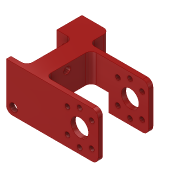
# Autodesk Inventor part: Odometry_Holder with motor clearance
Saved by Autodesk Inventor 2020 (Build 240168000, 168)
## iProperties
Created: 2019-06-02
Part Number: Odometry_Holder with motor clearance
Material: Generic
Document SubType Name: Modeling
Designer: ishaa
Density: 1 g/cm^3
Appearance: Default
Author: ishaa
Autodesk Inventor part; units mm, degrees
ref_plane "YZ Plane" through (0, 0, 0) normal (1, 0, 0) x (0, 1, 0)
ref_plane "XZ Plane" through (0, 0, 0) normal (0, 1, 0) x (-1, 0, 0)
ref_plane "XY Plane" through (0, 0, 0) normal (0, 0, 1) x (1, 0, 0)
sketch "Sketch1" plane through (0, 0, 0) normal (0, 1, 0) x (-1, 0, 0)
  line L0 (-8.3746, 16.5585) -> (42.4254, 16.5585)
  line L1 (42.4254, 16.5585) -> (42.4254, 14.0185)
  line L2 (42.4254, 14.0185) -> (33.5354, 14.0185)
  line L3 (33.5354, 14.0185) -> (33.5354, -11.3815)
  line L4 (33.5354, -11.3815) -> (42.4254, -11.3815)
  line L5 (42.4254, -11.3815) -> (42.4254, -13.9215)
  line L6 (42.4254, -13.9215) -> (-8.3746, -13.9215)
  line L7 (-8.3746, 16.5585) -> (-8.3746, 14.0185)
  line L8 (-8.3746, 14.0185) -> (23.3754, 14.0185)
  line L9 (23.3754, 14.0185) -> (23.3754, -11.3815)
  line L10 (23.3754, -11.3815) -> (-8.3746, -11.3815)
  line L11 (-8.3746, -11.3815) -> (-8.3746, -13.9215)
  point P0 (0, 0)
  dimension "d0" = 30.48
  dimension "d1" = 2.54
  dimension "d2" = 2.54
  dimension "d4" = 2.54
  dimension "d5" = 2.54
  dimension "d6" = 8.89
  dimension "d7" = 50.8
  dimension "d8" = 31.75
  constraints: 24 end point, 9 perpendicular, 3 point on line, 1 horizontal, 1 vertical
  measures "d0" distance between parallel lines of L0 L6
  measures "d1" distance between parallel lines of L8 L0
  measures "d2" distance between parallel lines of L6 L10
  measures "d4" distance between parallel lines of L2 L0
  measures "d5" distance between parallel lines of L6 L4
  measures "d6" distance of L1.end L2.end
  measures "d7" distance of L0.start L0.end
  measures "d8" distance of L7.end L8.end
extrude "Extrusion1" add sketch "Sketch1" along normal blind 25.4
sketch "Sketch4" plane through (8.3746, 0, -13.9215) normal (0, 0, -1) x (-1, 0, 0)
  line L0 (50.8, 0) -> (0, 0) projected
  line L1 (50.8, 0) -> (50.8, 25.4) projected
  line L2 (0, 25.4) -> (50.8, 25.4) projected
  line L3 (50.8, 25.4) -> (41.91, 25.4)
  line L4 (41.91, 25.4) -> (41.91, 0)
  line L5 (41.91, 0) -> (50.8, 0)
  line L6 (50.8, 0) -> (50.8, 25.4)
  point P0 (8.3746, 0)
  dimension "d56" = 8.89
  constraints: 8 end point, 2 parallel, 1 horizontal, 1 perpendicular, 1 point on line
  measures "d56" distance of L5.end L4.end
extrude "Extrusion3" add sketch "Sketch4" along normal blind 11.43
sketch "Sketch5" plane through (-42.4254, 0, 16.5585) normal (0, 0, 1) x (1, 0, 0)
  line L0 (50.8, 0) -> (50.8, 25.4) projected
  line L1 (50.8, 0) -> (0, 0) projected
  point P0 (40.64, 12.7)
  dimension "d11" = 10.16
  dimension "d12" = 12.7
  measures "d11" distance from line of L0 point (40.64, 12.7)
  measures "d12" distance from line of L1 point (40.64, 12.7)
hole "Hole1" at (-1.7854, 12.7, 16.5585) direction (0, 0, -1) diameter 9.779 end through all
sketch "Sketch6" plane through (-42.4254, 0, 16.5585) normal (0, 0, 1) x (1, 0, 0)
  line L0 (0, 0) -> (0, 25.4) projected
  line L1 (50.8, 0) -> (0, 0) projected
  point P0 (4, 4)
  dimension "d20" = 4
  dimension "d21" = 4
  measures "d20" distance from line of L0 point (4, 4)
  measures "d21" distance from line of L1 point (4, 4)
hole "Hole2" at (-38.4254, 4, 16.5585) direction (0, 0, -1) diameter 4.5 end through all
sketch "Sketch2" plane through (-42.4254, 0, 16.5585) normal (0, 0, 1) x (1, 0, 0)
  circle A0 centre (40.64, 12.7) radius 4.8895 projected
  line L0 (40.64, 22.225) -> (40.64, 3.175) construction
  circle A1 centre (40.64, 12.7) radius 4.8895 construction
  line L1 (40.64, 12.7) -> (33.9048, 19.4352) construction
  line L2 (40.64, 12.7) -> (33.9048, 5.9648) construction
  line L3 (40.64, 12.7) -> (47.3752, 5.9648) construction
  line L4 (40.64, 12.7) -> (47.3752, 19.4352) construction
  point P0 (42.4254, 0)
  dimension "d29" = 9.525
  dimension "d30" = 0
  dimension "d33" = 360
  dimension "d60" = 45
  dimension "d63" = 360
  constraints: 10 end point, 4 coincident, 16 other
  measures "d29" distance of A0.centre L0.end
  measures "d30" horizontal distance of A0.centre L0.end
  measures "d60" angle of L0 L1
hole "Hole3" at (-1.7854, 3.175, 16.5585) at (-1.7854, 22.225, 16.5585) at (-8.5206, 5.9648, 16.5585) at (-8.5206, 19.4352, 16.5585) at (4.9498, 19.4352, 16.5585) at (4.9498, 5.9648, 16.5585) direction (0, 0, -1) diameter 2.794 end through all
fillet "Fillet2" radius 3.175 8 edges at (-42.4254, 0, -18.3665) (-42.4254, 0, 15.2885) (-23.3754, 12.7, 14.0185) (-23.3754, 12.7, -11.3815) (8.3746, 0, -12.6515) (8.3746, 25.4, -12.6515) (8.3746, 25.4, 15.2885) (8.3746, 0, 15.2885)
hole "Hole4" at (-33.5354, 22.1488, 1.9535) direction (1, 0, 0) diameter 3.81 end through all
sketch "Sketch7" plane through (8.3746, 0, -25.3515) normal (0, 0, -1) x (-1, 0, 0)
  circle A0 centre (46.355, 19.1807) radius 1.524
  circle A1 centre (46.355, 12.5767) radius 1.524
  line L0 (50.8, 3.175) -> (50.8, 25.4) construction
  line L1 (41.91, 25.4) -> (41.91, 0) construction
  line L2 (50.8, 25.4) -> (41.91, 25.4) construction
  point P0 (8.3746, 0)
  dimension "d65" = 3.048
  dimension "d66" = 3.048
  dimension "d67" = 6.604
  dimension "d68" = 8.89
  dimension "d69" = 4.445
  dimension "d70" = 4.445
  dimension "d71" = 6.2193
  constraints: 2 centre point
  measures "d65" diameter of A0
  measures "d66" diameter of A1
  measures "d67" distance of A1.centre A0.centre
  measures "d68" distance between parallel lines of L1 L0
  measures "d69" distance from line of L0 A0.centre
  measures "d70" distance from line of L1 A1.centre
  measures "d71" distance from line of L2 A0.centre
extrude "Extrusion4" cut sketch "Sketch7" against normal up to surface (13.97 mm away)
sketch "Sketch8" plane through (-33.5354, 0, -11.3815) normal (-1, 0, 0) x (0, 0, 1)
  circle A0 centre (7.5184, -12.002) radius 17.9959 construction
  line L0 (-13.97, 3.175) -> (-13.97, 25.4) construction
  line L1 (-13.97, 6.25) -> (0, 6.25) construction
  line L2 (-13.97, 1.75) -> (0, 1.75) construction
  line L3 (0, 4.572) -> (0, 1.778) construction
  line L4 (0, 4) -> (-13.97, 4) construction
  line L5 (25.4, 0) -> (25.4, 3.175) projected
  line L6 (25.4, 0) -> (-11.43, 0)
  line L7 (-11.43, 0) -> (-11.43, 9.8039)
  line L8 (-11.43, 9.8039) -> (25.4, 9.8039)
  line L9 (25.4, 9.8039) -> (25.4, 0)
  point P0 (11.3815, 0)
  dimension "d74" = 35.9918
  dimension "d75" = 21.4884
  dimension "d76" = 4.5
  dimension "d77" = 2.25
  dimension "d78" = 16.002
  dimension "d79" = 2.54
  dimension "d80" = 21.8059
  constraints: 10 end point, 2 parallel, 2 perpendicular, 2 point on line, 1 centre point, 1 horizontal
  measures "d74" diameter of A0
  measures "d75" distance from line of L0 A0.centre
  measures "d76" distance between parallel lines of L1 L2
  measures "d77" distance between parallel lines of L2 L4
  measures "d78" distance from line of L4 A0.centre
  measures "d79" distance between parallel lines of L0 L7
  measures "d80" distance from line of A0.centre L8
extrude "Extrusion5" cut sketch "Sketch8" along normal blind 8.89 and the other way blind 19.8882
sketch "Sketch9" plane through (5.1996, 25.4, -13.9215) normal (0, 0, -1) x (-1, 0, 0)
  line L0 (0, 0) -> (38.735, 0) projected
  line L1 (18.8468, -15.5961) -> (38.735, -15.5961) projected
  line L2 (38.735, 0) -> (32.385, 0)
  line L3 (32.385, 0) -> (32.385, -15.5961)
  line L4 (32.385, -15.5961) -> (38.735, -15.5961)
  line L5 (38.735, -15.5961) -> (38.735, 0)
  point P0 (5.1996, -25.4)
  dimension "d85" = 6.35
  constraints: 8 end point, 2 parallel, 1 horizontal, 1 perpendicular, 1 point on line
  measures "d85" distance of L4.end L3.end
extrude "Extrusion6" add sketch "Sketch9" along normal up to surface (11.43 mm away)
fillet "Fillet3" radius 3.175 7 edges at (-27.1854, 17.6019, -13.9215) (-33.5354, 0, -24.0815) (-33.5354, 9.8039, -24.0815) (-33.5354, 17.602, -11.3815) (-33.5354, 17.602, 14.0185) (-26.8679, 9.8039, 14.0185) (-27.1854, 17.6019, -25.3515)
fillet "Fillet4" radius 3.175 1 edges at (-36.3929, 9.8039, -22.8115)
equation "\"d2\" = d1"
equation "\"d4\" = d1"
equation "\"d5\" = d1"
equation "\"d69\" = 0.5 * d68"
equation "\"d70\" = 0.5 * d68"
equation "\"d77\" = 0.5 * d76"
body "Solid1"
